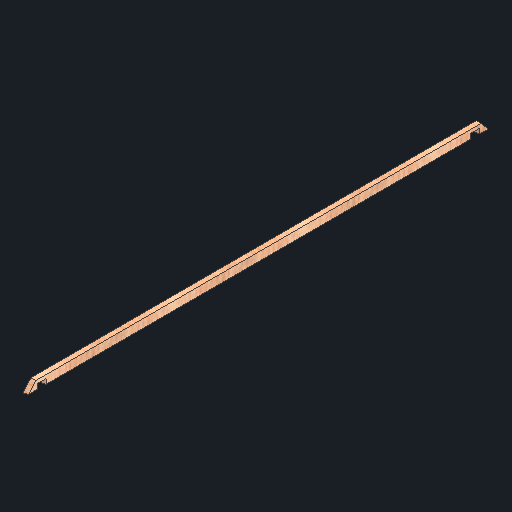
# Autodesk Inventor part: BASE_SIDEK_TREBUCHET
Saved by Autodesk Inventor 2026.2 (Build 302298010, 298A)
## iProperties
Created: 2026-02-18
Part Number: BASE_SIDEK_TREBUCHET
Material: Wood (Birch)
Document SubType Name: Modeling
Designer: 4aida
Density: 0.55 g/cm^3
Appearance: Birch - Natural Polished
Mass: 78.1862 g
Surface Area: 476.327 cm^2
Volume: 142.157 cm^3
Author: 4aida
Autodesk Inventor part; units mm, degrees
ref_plane "YZ Plane" through (0, 0, 0) normal (1, 0, 0) x (0, 1, 0)
ref_plane "XZ Plane" through (0, 0, 0) normal (0, 1, 0) x (-1, 0, 0)
ref_plane "XY Plane" through (0, 0, 0) normal (0, 0, 1) x (1, 0, 0)
sketch "Sketch1" plane through (0, 0, 0) normal (1, 0, 0) x (0, 1, 0)
  line L0 (-9.1281, -449.2848) -> (9.1281, -449.2848) construction
  line L1 (9.1281, -449.2848) -> (9.1281, 449.2848)
  line L2 (9.1281, 449.2848) -> (-9.1281, 449.2848) construction
  line L3 (-9.1281, 449.2848) -> (-9.1281, -449.2848)
  line L4 (-9.1281, -449.2848) -> (9.1281, 449.2848) construction
  line L5 (9.1281, -449.2848) -> (-9.1281, 449.2848) construction
  line L6 (-9.1281, 449.2848) -> (9.1281, 433.966)
  line L7 (-9.1281, -449.2848) -> (9.1281, -433.966)
  point P0 (0, 0)
  dimension "d0" = 898.5697
  dimension "d1" = 18.2563
  dimension "d16" = 40
  dimension "d17" = 40
  constraints: 16 end point, 2 midpoint, 2 parallel, 2 point on line, 1 horizontal, 1 perpendicular
  measures "d0" distance of L0.end L1.end
  measures "d1" distance of L1.end L2.end
  measures "d16" angle of L2 L6
  measures "d17" angle of L7 L0
extrude "Extrusion1" add sketch "Sketch1" along normal blind 9.525
chamfer "Chamfer1" distance 9.525 angle 11.388 1 edges at (9.525, -9.1281, 0) measured on face at (3.175, -9.1281, 149.7616)
sketch "Sketch4" plane through (0, -9.1281, -449.2848) normal (0.1975, -0.9803, 0) x (0.9803, 0.1975, 0)
  line L0 (0, 880.8231) -> (12.9422, 880.8231)
  line L1 (12.9422, 880.8231) -> (12.9422, 863.3606)
  line L2 (12.9422, 863.3606) -> (0, 863.3606)
  line L3 (0, 863.3606) -> (0, 880.8231)
  line L4 (12.9422, 15.3188) -> (12.9422, 883.2508) projected
  line L5 (0, 898.5697) -> (0, 0) projected
  point P0 (1.8024, 449.2848)
  dimension "d21" = 17.7466
  dimension "d22" = 17.4625
  constraints: 8 end point, 2 parallel, 2 point on line, 1 horizontal, 1 perpendicular
  measures "d21" distance from line of L0 L5.start
  measures "d22" distance of L2.end L0.start
extrude "Extrusion4" cut sketch "Sketch4" against normal blind 9.525
mirror "Mirror2" about plane through (0, 0, 0) normal (0, 0, 1) of "Extrusion4"
body "Solid1"
